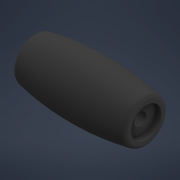
# Autodesk Inventor part: roller
Saved by Autodesk Inventor 2021.3 (Build 253353000, 353)
## iProperties
Created: 2021-10-17
Part Number: roller
Material: Rubber, Black
Document SubType Name: Modeling
Designer: ASUS
Density: 0.93 g/cm^3
Appearance: Rubber - Black
Author: ASUS
Autodesk Inventor part; units mm, degrees
ref_plane "YZ Plane" through (0, 0, 0) normal (1, 0, 0) x (0, 1, 0)
ref_plane "XZ Plane" through (0, 0, 0) normal (0, 1, 0) x (-1, 0, 0)
ref_plane "XY Plane" through (0, 0, 0) normal (0, 0, 1) x (1, 0, 0)
sketch "Sketch1" plane through (0, 0, 0) normal (0, 1, 0) x (-1, 0, 0)
  line L0 (0, 0) -> (-14, 0)
  line L1 (0, 0) -> (14, 0)
  line L2 (-14, 0) -> (-14, -5.25)
  line L3 (14, 0) -> (14, -5.25)
  arc A0 (-14, -5.25) -> (14, -5.25) centre (0, 61.6112) ccw
  line L4 (0, -6.7) -> (0, 0) construction
  dimension "d0" = 14
  dimension "d1" = 14
  dimension "d2" = 5.25
  dimension "d3" = 6.7
  constraints: 10 end point, 3 point on circle, 3 vertical, 2 horizontal, 1 centre point
  measures "d0" distance of L0.start L0.end
  measures "d1" distance of L0.start L1.end
  measures "d2" distance of L0.end L2.end
  measures "d3" distance of L4.start L0.start
revolve "Revolution1" add sketch "Sketch1" angle 360 about axis through (0, 0, 0) along (-1, 0, 0)
fillet "Fillet1" radius 1 2 edges at (14, 0, 5.25) (-14, 0, 5.25)
sketch "Sketch2" plane through (-14, 0, 0) normal (-1, 0, 0) x (0, 0, 1)
  circle A0 centre (0, 0) radius 3.75
  dimension "d6" = 7.5
  constraints: 1 centre point, 1 coincident
  measures "d6" diameter of A0
extrude "Extrusion1" cut sketch "Sketch2" against normal blind 1.5
mirror "Mirror1" about plane through (0, 0, 0) normal (1, 0, 0) of "Extrusion1"
sketch "Sketch3" plane through (12.5, 0, 0) normal (1, 0, 0) x (0, 0, -1)
  circle A0 centre (0, 0) radius 3.75 projected
  constraints: 1 coincident
hole "Hole1" at (12.5, 0, 0) direction (-1, 0, 0) diameter 3.015 end through all
body "Solid1"
